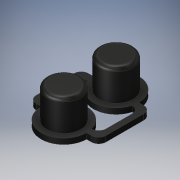
# Autodesk Inventor part: push_buttons
Saved by Autodesk Inventor 2017 (Build 210142000, 142)
## iProperties
Created: 2018-01-15
Part Number: push_buttons
Material: Generic
Document SubType Name: Modeling
Designer: Mitch
Density: 1 g/cm^3
Appearance: Glossy - Black
Author: Mitch
Autodesk Inventor part; units mm, degrees
ref_plane "YZ Plane" through (0, 0, 0) normal (1, 0, 0) x (0, 1, 0)
ref_plane "XZ Plane" through (0, 0, 0) normal (0, 1, 0) x (-1, 0, 0)
ref_plane "XY Plane" through (0, 0, 0) normal (0, 0, 1) x (1, 0, 0)
sketch "Sketch1" plane through (0, 0, 0) normal (0, 1, 0) x (-1, 0, 0)
  circle A0 centre (0, 0) radius 4.953
  circle A1 centre (0, -11.43) radius 4.953
  dimension "d0" = 9.906
  dimension "d1" = 9.906
  dimension "d2" = 11.43
  constraints: 2 centre point, 1 coincident
  measures "d0" diameter of A0
  measures "d1" diameter of A1
  measures "d2" distance of A1.centre A0.centre
extrude "Extrusion1" add sketch "Sketch1" along normal blind 1.2192
sketch "Sketch2" plane through (0, 1.2192, 0) normal (0, 1, 0) x (1, 0, 0)
  circle A0 centre (0, 0) radius 3.683
  circle A1 centre (0, 11.43) radius 3.683
  dimension "d5" = 7.366
  dimension "d6" = 7.366
  dimension "d7" = 11.43
  constraints: 2 centre point, 1 coincident
  measures "d5" diameter of A0
  measures "d6" diameter of A1
  measures "d7" distance of A0.centre A1.centre
extrude "Extrusion2" add sketch "Sketch2" along normal blind 6.731
fillet "Fillet1" radius 0.7937 2 edges at (-3.683, 7.9502, -11.43) (-3.683, 7.9502, 0)
sketch "Sketch3" plane through (0, 0, 0) normal (0, -1, 0) x (1, 0, 0)
  circle A0 centre (0, 0) radius 2.8892 projected
  line L0 (-4.953, 0) -> (-6.0325, 0)
  line L1 (-7.62, -1.5875) -> (-7.62, -9.8425)
  line L2 (-4.953, -11.43) -> (-6.0325, -11.43)
  circle A1 centre (0, -11.43) radius 4.953 projected
  line L3 (4.953, -11.4315) -> (6.039, -11.4309)
  line L4 (7.6256, -9.8425) -> (7.6209, -1.5873)
  line L5 (6.0334, -0.0007) -> (4.953, -0.0007)
  line L6 (-6.35, -8.5725) -> (-6.35, -2.8575)
  line L7 (-4.7625, -1.27) -> (-4.7874, -1.27)
  line L8 (-4.7874, -10.16) -> (-4.7625, -10.16)
  circle A2 centre (0, 0) radius 4.953 projected
  line L9 (4.7874, -1.27) -> (4.7641, -1.27)
  line L10 (6.3516, -2.8566) -> (6.3548, -8.5716)
  line L11 (4.7682, -10.16) -> (4.7874, -10.16)
  arc A3 (6.039, -11.4309) -> (7.6256, -9.8425) centre (6.0381, -9.8434) ccw
  arc A4 (4.7682, -10.16) -> (6.3548, -8.5716) centre (4.7673, -8.5725) ccw
  arc A5 (7.6209, -1.5873) -> (6.0334, -0.0007) centre (6.0334, -1.5882) ccw
  arc A6 (6.3516, -2.8566) -> (4.7641, -1.27) centre (4.7641, -2.8575) ccw
  arc A7 (-6.0325, 0) -> (-7.62, -1.5875) centre (-6.0325, -1.5875) ccw
  arc A8 (-4.7625, -1.27) -> (-6.35, -2.8575) centre (-4.7625, -2.8575) ccw
  arc A9 (-6.35, -8.5725) -> (-4.7625, -10.16) centre (-4.7625, -8.5725) ccw
  arc A10 (-7.62, -9.8425) -> (-6.0325, -11.43) centre (-6.0325, -9.8425) ccw
  circle A11 centre (0, -11.43) radius 2.8892 projected
  point P0 (7.6265, -11.43)
  dimension "d12" = 1.27
  dimension "d14" = 1.5875
  dimension "d17" = 7.62
  dimension "d18" = 1.27
  dimension "d21" = 7.62
  dimension "d22" = 1.27
  dimension "d23" = 1.2716
  constraints: 24 end point, 24 point on circle, 16 tangent, 8 centre point, 7 equal radius, 6 perpendicular, 3 point on line, 1 horizontal
  measures "d12" distance between parallel lines of L2 L8
  measures "d14" radius of A3
  measures "d17" distance from line of A1.centre L1
  measures "d18" distance between parallel lines of L1 L6
  measures "d21" distance from line of A0.centre L4
  measures "d22" distance between parallel lines of L10 L4
  measures "d23" distance between parallel lines of L3 L11
extrude "Extrusion3" add sketch "Sketch3" against normal blind 1.2192 contours A2 A8 L6 A9 A1 L2 A10 L1 A7 L0 | L5 A5 L4 A3 L3 A1 A4 L10 A6 A2
body "Solid1"
